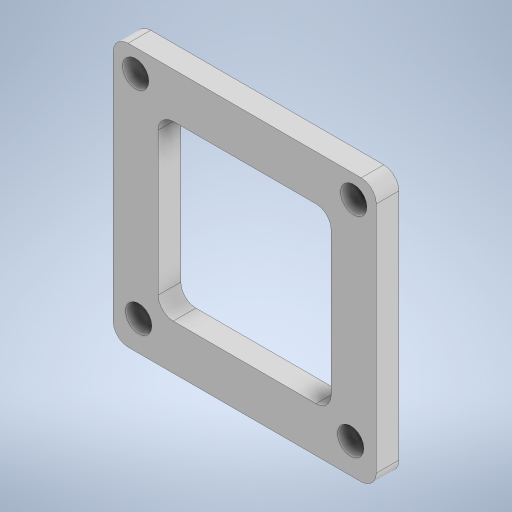
# Autodesk Inventor part: load_cell_frame
Saved by Autodesk Inventor 2024 (Build 280153000, 153)
## iProperties
Created: 2023-09-05
Part Number: load_cell_frame
Material: Generic
Document SubType Name: Modeling
Designer: Pintu
Density: 1 g/cm^3
Appearance: Default
Author: Pintu
Autodesk Inventor part; units mm, degrees
ref_plane "YZ Plane" through (0, 0, 0) normal (1, 0, 0) x (0, 1, 0)
ref_plane "XZ Plane" through (0, 0, 0) normal (0, 1, 0) x (-1, 0, 0)
ref_plane "XY Plane" through (0, 0, 0) normal (0, 0, 1) x (1, 0, 0)
sketch "Sketch1" plane through (0, 0, 0) normal (0, 0, 1) x (1, 0, 0)
  line L0 (-17.5, 17.5) -> (17.5, 17.5)
  line L1 (17.5, 17.5) -> (17.5, -17.5)
  line L2 (17.5, -17.5) -> (-17.5, -17.5)
  line L3 (-17.5, -17.5) -> (-17.5, 17.5)
  line L4 (-17.5, 17.5) -> (17.5, -17.5) construction
  line L5 (17.5, 17.5) -> (-17.5, -17.5) construction
  circle A0 centre (-14.5, 14.5) radius 1.75
  circle A1 centre (-14.0979, -13.5) radius 1.75
  line L6 (0, 17.5) -> (0, -17.5) construction
  line L7 (17.5, -17.5) -> (17.5, 17.5)
  circle A2 centre (14.5, 14.5) radius 1.75
  circle A3 centre (14.0979, -13.5) radius 1.75
  line L8 (-11.5, 11.5) -> (11.5, 11.5)
  line L9 (11.5, 11.5) -> (11.5, -11.5)
  line L10 (11.5, -11.5) -> (-11.5, -11.5)
  line L11 (-11.5, -11.5) -> (-11.5, 11.5)
  line L12 (-11.5, 11.5) -> (11.5, -11.5) construction
  line L13 (11.5, 11.5) -> (-11.5, -11.5) construction
  point P0 (0, 0)
  dimension "d0" = 35
  dimension "d1" = 35
  dimension "d3" = 3.5
  dimension "d4" = 3.5
  dimension "d5" = 28
  dimension "d6" = 3
  dimension "d7" = 3
  dimension "d9" = 23
  dimension "d10" = 23
  constraints: 28 end point, 6 midpoint, 4 centre point, 4 parallel, 2 horizontal, 2 perpendicular, 2 symmetric about line, 2 other
  measures "d0" distance of L1.end L2.end
  measures "d1" distance of L0.end L1.end
  measures "d3" diameter of A0
  measures "d4" diameter of A1
  measures "d5" vertical distance of A1.centre A0.centre
  measures "d6" distance from line of L0 A0.centre
  measures "d7" distance from line of L3 A0.centre
  measures "d9" distance of L9.end L10.end
  measures "d10" distance of L8.end L9.end
extrude "Extrusion1" add sketch "Sketch1" along normal blind 3
fillet "Fillet1" radius 2 8 edges at (-11.5, 11.5, 1.5) (-11.5, -11.5, 1.5) (11.5, -11.5, 1.5) (11.5, 11.5, 1.5) (-17.5, -17.5, 1.5) (17.5, -17.5, 1.5) (-17.5, 17.5, 1.5) (17.5, 17.5, 1.5)
body "Solid1"
